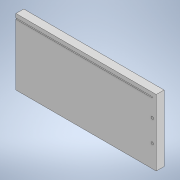
# Autodesk Inventor part: CubeBase
Saved by Autodesk Inventor 2020 (Build 240168000, 168)
## iProperties
Created: 2019-12-01
Part Number: CubeBase
Material: Generic
Document SubType Name: Modeling
Designer: torto
Density: 1 g/cm^3
Appearance: Default
Author: torto
Autodesk Inventor part; units mm, degrees
ref_plane "YZ Plane" through (0, 0, 0) normal (1, 0, 0) x (0, 1, 0)
ref_plane "XZ Plane" through (0, 0, 0) normal (0, 1, 0) x (-1, 0, 0)
ref_plane "XY Plane" through (0, 0, 0) normal (0, 0, 1) x (1, 0, 0)
sketch "Sketch1" plane through (0, 0, 0) normal (0, 0, 1) x (1, 0, 0)
  line L0 (0, 0) -> (228.6, 0)
  line L1 (228.6, 0) -> (228.6, 107.95)
  line L2 (228.6, 107.95) -> (0, 107.95)
  line L3 (0, 107.95) -> (0, 0)
  line L4 (228.6, 107.95) -> (222.25, 107.95) construction
  line L5 (222.25, 107.95) -> (222.25, 101.6) construction
  line L6 (222.25, 101.6) -> (228.6, 101.6) construction
  line L7 (228.6, 101.6) -> (228.6, 107.95) construction
  line L8 (222.25, 101.6) -> (0, 101.6)
  line L9 (0, 101.6) -> (0, 100.076)
  line L10 (0, 100.076) -> (222.25, 100.076)
  line L11 (222.25, 100.076) -> (222.25, 101.6)
  line L12 (228.6, 0) -> (222.25, 0) construction
  line L13 (222.25, 0) -> (222.25, 35.9833) construction
  line L14 (222.25, 35.9833) -> (228.6, 35.9833) construction
  line L15 (228.6, 35.9833) -> (228.6, 0) construction
  circle A0 centre (222.25, 35.9833) radius 2
  circle A1 centre (222.25, 71.9667) radius 2
  dimension "length" = 228.6
  dimension "height" = 107.95
  dimension "d3" = 6.35
  dimension "d4" = 6.35
  dimension "d5" = 222.25
  dimension "d6" = 1.524
  dimension "spacing" = 35.9833
  dimension "d9" = 6.35
  dimension "d10" = 4
  dimension "d13" = 35.9833
  constraints: 32 end point, 8 parallel, 4 horizontal, 4 perpendicular, 2 centre point, 2 coincident, 1 vertical, 3 other
  measures "length" distance of L2.end L1.end
  measures "height" distance of L1.end L0.end
  measures "d3" distance of L5.end L4.end
  measures "d4" distance of L5.end L6.end
  measures "d5" distance of L10.end L9.end
  measures "d6" distance of L9.end L8.end
  measures "spacing" distance of L12.end L13.end
  measures "d9" distance of L13.end L14.end
  measures "d10" diameter of A0
  measures "d13" distance of A0.centre A1.centre
extrude "Generic Shape" add sketch "Sketch1" along normal blind 12.7
sketch "Sketch2" plane through (0, 0, 12.7) normal (0, 0, 1) x (1, 0, 0)
  line L0 (228.6, 107.95) -> (0, 107.95) construction
  line L1 (228.6, 107.95) -> (222.25, 107.95) construction
  line L2 (222.25, 107.95) -> (222.25, 101.6) construction
  line L3 (222.25, 101.6) -> (228.6, 101.6) construction
  line L4 (228.6, 101.6) -> (228.6, 107.95) construction
  line L5 (222.25, 101.6) -> (0, 101.6)
  line L6 (0, 101.6) -> (0, 100.076)
  line L7 (0, 100.076) -> (222.25, 100.076)
  line L8 (222.25, 100.076) -> (222.25, 101.6)
  point P0 (0, 0)
  dimension "d21" = 6.35
  dimension "d22" = 6.35
  dimension "d23" = 222.25
  dimension "d24" = 1.524
  constraints: 16 end point, 4 parallel, 2 horizontal, 2 perpendicular
  measures "d21" distance of L2.end L1.end
  measures "d22" distance of L2.end L3.end
  measures "d23" distance of L7.end L6.end
  measures "d24" distance of L6.end L5.end
extrude "PCB Notch" cut sketch "Sketch2" against normal blind 6.35
sketch "Sketch4" plane through (0, 0, 0) normal (-1, 0, 0) x (0, 0, 1)
  line L0 (0, 0) -> (6.35, 0) construction
  line L1 (6.35, 0) -> (6.35, 35.9833) construction
  line L2 (6.35, 35.9833) -> (0, 35.9833) construction
  line L3 (0, 35.9833) -> (0, 0) construction
  circle A0 centre (6.35, 35.9833) radius 2
  line L4 (0, 107.95) -> (6.35, 107.95) construction
  line L5 (6.35, 107.95) -> (6.35, 71.9667) construction
  line L6 (6.35, 71.9667) -> (0, 71.9667) construction
  line L7 (0, 71.9667) -> (0, 107.95) construction
  circle A1 centre (6.35, 71.9667) radius 2
  dimension "d33" = 6.35
  dimension "d34" = 35.9833
  dimension "ScrewDiameter" = 4
  dimension "d36" = 6.35
  dimension "d37" = 35.9833
  dimension "d38" = 4
  constraints: 16 end point, 4 parallel, 2 centre point, 2 coincident, 2 horizontal, 2 perpendicular
  measures "d33" distance of L2.end L1.end
  measures "d34" distance of L1.end L0.end
  measures "ScrewDiameter" diameter of A0
  measures "d36" distance of L5.end L6.end
  measures "d37" distance of L4.end L5.end
  measures "d38" diameter of A1
extrude "2in Screw Depth" cut sketch "Sketch4" against normal blind 50.8
equation "\"d3\" = 0.5 * thickness"
equation "\"d4\" = 0.5 * thickness"
equation "\"d5\" = length - 0.5 * thickness"
equation "\"spacing\" = 0.333333 * height"
equation "\"d9\" = 0.5 * thickness"
equation "\"d10\" = ScrewDiameter"
equation "\"d13\" = spacing"
equation "\"d25\" = 0.5 * thickness"
equation "\"d33\" = 0.5 * thickness"
equation "\"d34\" = 0.333333 * height"
equation "\"d36\" = 0.5 * thickness"
equation "\"d37\" = 0.333333 * height"
equation "\"d38\" = ScrewDiameter"
equation "\"thickness\" = 12.7"
body "Solid1"
